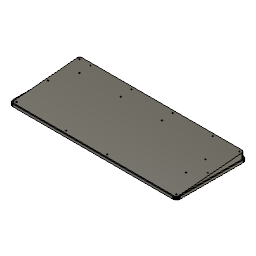
Base (Autodesk Fusion 360 design; units mm, degrees)
part number: 2026-06-20-14-02-00-105
Autodesk Fusion 360 part; units mm, degrees
note: some values were not read from the file. Chosen so that the rebuilt part matches the saved one: which pieces of a blend or face edit are solid.
(part 1 of 4)
imported_body "Derived Base Feature1" makes body 1
sketch "Sketch1" plane through (0, 0, 0) normal (0, 0, 1) x (1, 0, 0)
  line L0 (324.2389, -5.001) -> (324.612, -5.015)
  line L1 (324.612, -5.015) -> (324.9851, -5.059)
  line L2 (324.9851, -5.059) -> (325.3502, -5.132)
  line L3 (325.3502, -5.132) -> (325.71, -5.234)
  line L4 (325.71, -5.234) -> (326.0619, -5.363)
  line L5 (326.0619, -5.363) -> (326.4006, -5.52)
  line L6 (326.4006, -5.52) -> (326.726, -5.702)
  line L7 (326.726, -5.702) -> (327.0382, -5.91)
  line L8 (327.0382, -5.91) -> (327.3319, -6.142)
  line L9 (327.3319, -6.142) -> (327.6071, -6.395)
  line L10 (327.6071, -6.395) -> (327.8611, -6.67)
  line L11 (327.8611, -6.67) -> (328.0913, -6.964)
  line L12 (328.0913, -6.964) -> (328.3003, -7.275)
  line L13 (328.3003, -7.275) -> (328.4829, -7.601)
  line L14 (328.4829, -7.601) -> (328.639, -7.94)
  line L15 (328.639, -7.94) -> (328.7686, -8.291)
  line L16 (328.7686, -8.291) -> (328.8691, -8.651)
  line L17 (328.8691, -8.651) -> (328.9432, -9.018)
  line L18 (328.9432, -9.018) -> (328.9882, -9.389)
  line L19 (328.9882, -9.389) -> (329.0014, -9.763)
  line L20 (329.0014, -9.763) -> (329.0014, -133.7389)
  line L21 (329.0014, -133.7389) -> (328.9882, -134.1131)
  line L22 (328.9882, -134.1131) -> (328.9432, -134.484)
  line L23 (328.9432, -134.484) -> (328.8691, -134.851)
  line L24 (328.8691, -134.851) -> (328.7686, -135.2111)
  line L25 (328.7686, -135.2111) -> (328.639, -135.5619)
  line L26 (328.639, -135.5619) -> (328.4829, -135.9011)
  line L27 (328.4829, -135.9011) -> (328.3003, -136.2271)
  line L28 (328.3003, -136.2271) -> (328.0913, -136.538)
  line L29 (328.0913, -136.538) -> (327.8611, -136.8319)
  line L30 (327.8611, -136.8319) -> (327.6071, -137.1071)
  line L31 (327.6071, -137.1071) -> (327.3319, -137.36)
  line L32 (327.3319, -137.36) -> (327.0382, -137.5921)
  line L33 (327.0382, -137.5921) -> (326.726, -137.8)
  line L34 (326.726, -137.8) -> (326.4006, -137.9821)
  line L35 (326.4006, -137.9821) -> (326.0619, -138.139)
  line L36 (326.0619, -138.139) -> (325.71, -138.2681)
  line L37 (325.71, -138.2681) -> (325.3502, -138.3699)
  line L38 (325.3502, -138.3699) -> (324.9851, -138.443)
  line L39 (324.9851, -138.443) -> (324.612, -138.4869)
  line L40 (324.612, -138.4869) -> (324.2389, -138.502)
  line L41 (324.2389, -138.502) -> (9.763, -138.5009)
  line L42 (9.763, -138.5009) -> (9.389, -138.4869)
  line L43 (9.389, -138.4869) -> (9.018, -138.443)
  line L44 (9.018, -138.443) -> (8.651, -138.3699)
  line L45 (8.651, -138.3699) -> (8.291, -138.2681)
  line L46 (8.291, -138.2681) -> (7.94, -138.139)
  line L47 (7.94, -138.139) -> (7.601, -137.9821)
  line L48 (7.601, -137.9821) -> (7.275, -137.8)
  line L49 (7.275, -137.8) -> (6.964, -137.5921)
  line L50 (6.964, -137.5921) -> (6.67, -137.36)
  line L51 (6.67, -137.36) -> (6.395, -137.1071)
  line L52 (6.395, -137.1071) -> (6.142, -136.8319)
  line L53 (6.142, -136.8319) -> (5.91, -136.538)
  line L54 (5.91, -136.538) -> (5.702, -136.2271)
  line L55 (5.702, -136.2271) -> (5.52, -135.9011)
  line L56 (5.52, -135.9011) -> (5.363, -135.5619)
  line L57 (5.363, -135.5619) -> (5.234, -135.2111)
  line L58 (5.234, -135.2111) -> (5.132, -134.851)
  line L59 (5.132, -134.851) -> (5.059, -134.484)
  line L60 (5.059, -134.484) -> (5.015, -134.1131)
  line L61 (5.015, -134.1131) -> (5, -133.7389)
  line L62 (5, -133.7389) -> (5.001, -9.763)
  line L63 (5.001, -9.763) -> (5.015, -9.389)
  line L64 (5.015, -9.389) -> (5.059, -9.018)
  line L65 (5.059, -9.018) -> (5.132, -8.651)
  line L66 (5.132, -8.651) -> (5.234, -8.291)
  line L67 (5.234, -8.291) -> (5.363, -7.94)
  line L68 (5.363, -7.94) -> (5.52, -7.601)
  line L69 (5.52, -7.601) -> (5.702, -7.275)
  line L70 (5.702, -7.275) -> (5.91, -6.964)
  line L71 (5.91, -6.964) -> (6.142, -6.67)
  line L72 (6.142, -6.67) -> (6.395, -6.395)
  line L73 (6.395, -6.395) -> (6.67, -6.142)
  line L74 (6.67, -6.142) -> (6.964, -5.91)
  line L75 (6.964, -5.91) -> (7.275, -5.702)
  line L76 (7.275, -5.702) -> (7.601, -5.52)
  line L77 (7.601, -5.52) -> (7.94, -5.363)
  line L78 (7.94, -5.363) -> (8.291, -5.234)
  line L79 (8.291, -5.234) -> (8.651, -5.132)
  line L80 (8.651, -5.132) -> (9.018, -5.059)
  line L81 (9.018, -5.059) -> (9.389, -5.015)
  line L82 (9.389, -5.015) -> (9.763, -5)
  line L83 (9.763, -5) -> (324.2389, -5.001)
  line L84 (324.2654, -5.0281) -> (324.6411, -5.0421)
  line L85 (324.6411, -5.0421) -> (325.0115, -5.0861)
  line L86 (325.0115, -5.0861) -> (325.3793, -5.1591)
  line L87 (325.3793, -5.1591) -> (325.7391, -5.2611)
  line L88 (325.7391, -5.2611) -> (326.0884, -5.3901)
  line L89 (326.0884, -5.3901) -> (326.427, -5.5471)
  line L90 (326.427, -5.5471) -> (326.7551, -5.7291)
  line L91 (326.7551, -5.7291) -> (327.0647, -5.9371)
  line L92 (327.0647, -5.9371) -> (327.3584, -6.1691)
  line L93 (327.3584, -6.1691) -> (327.6336, -6.4221)
  line L94 (327.6336, -6.4221) -> (327.8875, -6.6971)
  line L95 (327.8875, -6.6971) -> (328.1204, -6.9911)
  line L96 (328.1204, -6.9911) -> (328.3268, -7.3021)
  line L97 (328.3268, -7.3021) -> (328.5093, -7.6281)
  line L98 (328.5093, -7.6281) -> (328.6654, -7.9671)
  line L99 (328.6654, -7.9671) -> (328.795, -8.3181)
  line L100 (328.795, -8.3181) -> (328.8982, -8.6781)
  line L101 (328.8982, -8.6781) -> (328.9697, -9.0451)
  line L102 (328.9697, -9.0451) -> (329.0147, -9.4161)
  line L103 (329.0147, -9.4161) -> (329.0279, -9.7901)
  line L104 (329.0279, -9.7901) -> (329.0279, -133.7662)
  line L105 (329.0279, -133.7662) -> (329.0147, -134.14)
  line L106 (329.0147, -134.14) -> (328.9697, -134.511)
  line L107 (328.9697, -134.511) -> (328.8982, -134.878)
  line L108 (328.8982, -134.878) -> (328.795, -135.2381)
  line L109 (328.795, -135.2381) -> (328.6654, -135.5892)
  line L110 (328.6654, -135.5892) -> (328.5093, -135.9281)
  line L111 (328.5093, -135.9281) -> (328.3268, -136.2541)
  line L112 (328.3268, -136.2541) -> (328.1204, -136.565)
  line L113 (328.1204, -136.565) -> (327.8875, -136.8592)
  line L114 (327.8875, -136.8592) -> (327.6336, -137.1341)
  line L115 (327.6336, -137.1341) -> (327.3584, -137.387)
  line L116 (327.3584, -137.387) -> (327.0647, -137.6191)
  line L117 (327.0647, -137.6191) -> (326.7551, -137.827)
  line L118 (326.7551, -137.827) -> (326.427, -138.0091)
  line L119 (326.427, -138.0091) -> (326.0884, -138.1662)
  line L120 (326.0884, -138.1662) -> (325.7391, -138.2951)
  line L121 (325.7391, -138.2951) -> (325.3793, -138.3972)
  line L122 (325.3793, -138.3972) -> (325.0115, -138.47)
  line L123 (325.0115, -138.47) -> (324.6411, -138.5141)
  line L124 (324.6411, -138.5141) -> (324.2654, -138.5289)
  line L125 (324.2654, -138.5289) -> (9.7901, -138.5282)
  line L126 (9.7901, -138.5282) -> (9.4161, -138.5141)
  line L127 (9.4161, -138.5141) -> (9.0451, -138.47)
  line L128 (9.0451, -138.47) -> (8.6781, -138.3972)
  line L129 (8.6781, -138.3972) -> (8.3181, -138.2951)
  line L130 (8.3181, -138.2951) -> (7.9671, -138.1662)
  line L131 (7.9671, -138.1662) -> (7.6281, -138.0091)
  line L132 (7.6281, -138.0091) -> (7.3021, -137.827)
  line L133 (7.3021, -137.827) -> (6.9911, -137.6191)
  line L134 (6.9911, -137.6191) -> (6.6971, -137.387)
  line L135 (6.6971, -137.387) -> (6.4221, -137.1341)
  line L136 (6.4221, -137.1341) -> (6.1691, -136.8592)
  line L137 (6.1691, -136.8592) -> (5.9371, -136.565)
  line L138 (5.9371, -136.565) -> (5.7291, -136.2541)
  line L139 (5.7291, -136.2541) -> (5.5471, -135.9281)
  line L140 (5.5471, -135.9281) -> (5.3901, -135.5892)
  line L141 (5.3901, -135.5892) -> (5.2611, -135.2381)
  line L142 (5.2611, -135.2381) -> (5.1591, -134.878)
  line L143 (5.1591, -134.878) -> (5.0861, -134.511)
  line L144 (5.0861, -134.511) -> (5.0421, -134.14)
  line L145 (5.0421, -134.14) -> (5.0271, -133.7662)
  line L146 (5.0271, -133.7662) -> (5.0281, -9.7901)
  line L147 (5.0281, -9.7901) -> (5.0421, -9.4161)
  line L148 (5.0421, -9.4161) -> (5.0861, -9.0451)
  line L149 (5.0861, -9.0451) -> (5.1591, -8.6781)
  line L150 (5.1591, -8.6781) -> (5.2611, -8.3181)
  line L151 (5.2611, -8.3181) -> (5.3901, -7.9671)
  line L152 (5.3901, -7.9671) -> (5.5471, -7.6281)
  line L153 (5.5471, -7.6281) -> (5.7291, -7.3021)
  line L154 (5.7291, -7.3021) -> (5.9371, -6.9911)
  line L155 (5.9371, -6.9911) -> (6.1691, -6.6971)
  line L156 (6.1691, -6.6971) -> (6.4221, -6.4221)
  line L157 (6.4221, -6.4221) -> (6.6971, -6.1691)
  line L158 (6.6971, -6.1691) -> (6.9911, -5.9371)
  line L159 (6.9911, -5.9371) -> (7.3021, -5.7291)
  line L160 (7.3021, -5.7291) -> (7.6281, -5.5471)
  line L161 (7.6281, -5.5471) -> (7.9671, -5.3901)
  line L162 (7.9671, -5.3901) -> (8.3181, -5.2611)
  line L163 (8.3181, -5.2611) -> (8.6781, -5.1591)
  line L164 (8.6781, -5.1591) -> (9.0451, -5.0861)
  line L165 (9.0451, -5.0861) -> (9.4161, -5.0421)
  line L166 (9.4161, -5.0421) -> (9.7901, -5.0271)
  line L167 (9.7901, -5.0271) -> (324.2654, -5.0281)
  line L168 (9.9401, -9.9401) -> (9.9401, -133.6162)
  line L169 (9.9401, -133.6162) -> (324.1172, -133.6162)
  line L170 (324.1172, -133.6162) -> (324.1172, -9.9401)
  line L171 (324.1172, -9.9401) -> (9.9401, -9.9401)
  line L172 (8.9397, -4.5648) -> (9.3495, -4.5162)
  line L173 (9.3495, -4.5162) -> (9.753, -4.5)
  line L174 (9.753, -4.5) -> (324.2483, -4.501)
  line L175 (324.2483, -4.501) -> (324.6507, -4.5161)
  line L176 (324.6507, -4.5161) -> (325.0635, -4.5648)
  line L177 (325.0635, -4.5648) -> (325.4676, -4.6456)
  line L178 (325.4676, -4.6456) -> (325.8645, -4.7581)
  line L179 (325.8645, -4.7581) -> (326.2534, -4.9007)
  line L180 (326.2534, -4.9007) -> (326.6281, -5.0744)
  line L181 (326.6281, -5.0744) -> (326.987, -5.2751)
  line L182 (326.987, -5.2751) -> (327.3323, -5.5051)
  line L183 (327.3323, -5.5051) -> (327.6566, -5.7613)
  line L184 (327.6566, -5.7613) -> (327.9605, -6.0408)
  line L185 (327.9605, -6.0408) -> (328.2422, -6.3457)
  line L186 (328.2422, -6.3457) -> (328.4962, -6.67)
  line L187 (328.4962, -6.67) -> (328.7266, -7.013)
  line L188 (328.7266, -7.013) -> (328.9288, -7.3739)
  line L189 (328.9288, -7.3739) -> (329.1012, -7.7485)
  line L190 (329.1012, -7.7485) -> (329.2447, -8.1369)
  line L191 (329.2447, -8.1369) -> (329.3556, -8.5341)
  line L192 (329.3556, -8.5341) -> (329.4372, -8.9383)
  line L193 (329.4372, -8.9383) -> (329.4872, -9.35)
  line L194 (329.4872, -9.35) -> (329.5014, -9.7542)
  line L195 (329.5014, -9.7542) -> (329.5014, -133.7478)
  line L196 (329.5014, -133.7478) -> (329.4872, -134.1521)
  line L197 (329.4872, -134.1521) -> (329.4372, -134.5637)
  line L198 (329.4372, -134.5637) -> (329.3556, -134.9678)
  line L199 (329.3556, -134.9678) -> (329.2447, -135.3652)
  line L200 (329.2447, -135.3652) -> (329.1013, -135.7534)
  line L201 (329.1013, -135.7534) -> (328.9288, -136.1282)
  line L202 (328.9288, -136.1282) -> (328.7266, -136.4892)
  line L203 (328.7266, -136.4892) -> (328.4961, -136.832)
  line L204 (328.4961, -136.832) -> (328.2422, -137.1562)
  line L205 (328.2422, -137.1562) -> (327.9606, -137.4613)
  line L206 (327.9606, -137.4613) -> (327.6566, -137.7408)
  line L207 (327.6566, -137.7408) -> (327.3323, -137.997)
  line L208 (327.3323, -137.997) -> (326.987, -138.2269)
  line L209 (326.987, -138.2269) -> (326.6281, -138.4277)
  line L210 (326.6281, -138.4277) -> (326.2534, -138.6013)
  line L211 (326.2534, -138.6013) -> (325.8645, -138.744)
  line L212 (325.8645, -138.744) -> (325.4675, -138.8564)
  line L213 (325.4675, -138.8564) -> (325.0635, -138.9372)
  line L214 (325.0635, -138.9372) -> (324.6514, -138.9857)
  line L215 (324.6514, -138.9857) -> (324.249, -139.002)
  line L216 (324.249, -139.002) -> (9.7536, -139.0009)
  line L217 (9.7536, -139.0009) -> (9.3502, -138.9858)
  line L218 (9.3502, -138.9858) -> (8.9397, -138.9372)
  line L219 (8.9397, -138.9372) -> (8.534, -138.8565)
  line L220 (8.534, -138.8565) -> (8.1364, -138.744)
  line L221 (8.1364, -138.744) -> (7.7484, -138.6012)
  line L222 (7.7484, -138.6012) -> (7.3738, -138.4279)
  line L223 (7.3738, -138.4279) -> (7.0137, -138.2268)
  line L224 (7.0137, -138.2268) -> (6.6697, -137.9968)
  line L225 (6.6697, -137.9968) -> (6.3454, -137.7408)
  line L226 (6.3454, -137.7408) -> (6.0411, -137.4609)
  line L227 (6.0411, -137.4609) -> (5.7612, -137.1565)
  line L228 (5.7612, -137.1565) -> (5.5054, -136.8323)
  line L229 (5.5054, -136.8323) -> (5.2752, -136.4884)
  line L230 (5.2752, -136.4884) -> (5.0742, -136.1283)
  line L231 (5.0742, -136.1283) -> (4.9007, -135.7535)
  line L232 (4.9007, -135.7535) -> (4.7581, -135.3657)
  line L233 (4.7581, -135.3657) -> (4.6455, -134.9681)
  line L234 (4.6455, -134.9681) -> (4.5648, -134.5623)
  line L235 (4.5648, -134.5623) -> (4.5162, -134.1526)
  line L236 (4.5162, -134.1526) -> (4.5, -133.749)
  line L237 (4.5, -133.749) -> (4.501, -9.7536)
  line L238 (4.501, -9.7536) -> (4.5161, -9.3501)
  line L239 (4.5161, -9.3501) -> (4.5648, -8.9397)
  line L240 (4.5648, -8.9397) -> (4.6455, -8.5339)
  line L241 (4.6455, -8.5339) -> (4.7581, -8.1364)
  line L242 (4.7581, -8.1364) -> (4.9007, -7.7484)
  line L243 (4.9007, -7.7484) -> (5.0742, -7.3738)
  line L244 (5.0742, -7.3738) -> (5.2752, -7.0137)
  line L245 (5.2752, -7.0137) -> (5.5053, -6.6697)
  line L246 (5.5053, -6.6697) -> (5.7612, -6.3454)
  line L247 (5.7612, -6.3454) -> (6.0411, -6.0411)
  line L248 (6.0411, -6.0411) -> (6.3454, -5.7612)
  line L249 (6.3454, -5.7612) -> (6.6697, -5.5053)
  line L250 (6.6697, -5.5053) -> (7.0137, -5.2752)
  line L251 (7.0137, -5.2752) -> (7.3737, -5.0742)
  line L252 (7.3737, -5.0742) -> (7.7484, -4.9007)
  line L253 (7.7484, -4.9007) -> (8.1364, -4.7581)
  line L254 (8.1364, -4.7581) -> (8.5339, -4.6455)
  line L255 (8.5339, -4.6455) -> (8.9397, -4.5648)
  line L256 (6.4647, -3.2911) -> (6.9819, -3.0516)
  line L257 (6.9819, -3.0516) -> (7.5179, -2.8546)
  line L258 (7.5179, -2.8546) -> (8.0654, -2.6995)
  line L259 (8.0654, -2.6995) -> (8.6263, -2.5879)
  line L260 (8.6263, -2.5879) -> (9.1914, -2.5209)
  line L261 (9.1914, -2.5209) -> (9.7129, -2.5)
  line L262 (9.7129, -2.5) -> (324.2858, -2.501)
  line L263 (324.2858, -2.501) -> (324.8056, -2.5205)
  line L264 (324.8056, -2.5205) -> (325.3772, -2.5879)
  line L265 (325.3772, -2.5879) -> (325.9371, -2.6999)
  line L266 (325.9371, -2.6999) -> (326.4823, -2.8544)
  line L267 (326.4823, -2.8544) -> (327.0195, -3.0513)
  line L268 (327.0195, -3.0513) -> (327.5381, -3.2918)
  line L269 (327.5381, -3.2918) -> (328.0311, -3.5675)
  line L270 (328.0311, -3.5675) -> (328.5085, -3.8855)
  line L271 (328.5085, -3.8855) -> (328.9551, -4.2384)
  line L272 (328.9551, -4.2384) -> (329.3743, -4.6238)
  line L273 (329.3743, -4.6238) -> (329.7667, -5.0485)
  line L274 (329.7667, -5.0485) -> (330.1156, -5.4942)
  line L275 (330.1156, -5.4942) -> (330.4319, -5.9649)
  line L276 (330.4319, -5.9649) -> (330.7124, -6.4656)
  line L277 (330.7124, -6.4656) -> (330.9504, -6.9827)
  line L278 (330.9504, -6.9827) -> (331.149, -7.5204)
  line L279 (331.149, -7.5204) -> (331.3016, -8.0666)
  line L280 (331.3016, -8.0666) -> (331.4132, -8.6195)
  line L281 (331.4132, -8.6195) -> (331.4829, -9.194)
  line L282 (331.4829, -9.194) -> (331.5014, -9.7189)
  line L283 (331.5014, -9.7189) -> (331.5014, -133.7831)
  line L284 (331.5014, -133.7831) -> (331.4829, -134.308)
  line L285 (331.4829, -134.308) -> (331.4132, -134.8825)
  line L286 (331.4132, -134.8825) -> (331.3016, -135.4353)
  line L287 (331.3016, -135.4353) -> (331.149, -135.9818)
  line L288 (331.149, -135.9818) -> (330.9504, -136.5192)
  line L289 (330.9504, -136.5192) -> (330.7125, -137.0363)
  line L290 (330.7125, -137.0363) -> (330.4317, -137.5375)
  line L291 (330.4317, -137.5375) -> (330.1155, -138.008)
  line L292 (330.1155, -138.008) -> (329.7669, -138.4531)
  line L293 (329.7669, -138.4531) -> (329.3745, -138.8782)
  line L294 (329.3745, -138.8782) -> (328.9551, -139.2637)
  line L295 (328.9551, -139.2637) -> (328.5085, -139.6166)
  line L296 (328.5085, -139.6166) -> (328.0312, -139.9345)
  line L297 (328.0312, -139.9345) -> (327.5379, -140.2104)
  line L298 (327.5379, -140.2104) -> (327.0196, -140.4505)
  line L299 (327.0196, -140.4505) -> (326.4822, -140.6477)
  line L300 (326.4822, -140.6477) -> (325.9367, -140.8021)
  line L301 (325.9367, -140.8021) -> (325.377, -140.9141)
  line L302 (325.377, -140.9141) -> (324.8089, -140.981)
  line L303 (324.8089, -140.981) -> (324.2894, -141.002)
  line L304 (324.2894, -141.002) -> (9.7161, -141.0009)
  line L305 (9.7161, -141.0009) -> (9.1949, -140.9814)
  line L306 (9.1949, -140.9814) -> (8.6265, -140.9141)
  line L307 (8.6265, -140.9141) -> (8.0658, -140.8025)
  line L308 (8.0658, -140.8025) -> (7.5179, -140.6475)
  line L309 (7.5179, -140.6475) -> (6.9818, -140.4503)
  line L310 (6.9818, -140.4503) -> (6.4649, -140.211)
  line L311 (6.4649, -140.211) -> (5.9687, -139.9339)
  line L312 (5.9687, -139.9339) -> (5.4925, -139.6155)
  line L313 (5.4925, -139.6155) -> (5.047, -139.2639)
  line L314 (5.047, -139.2639) -> (4.6255, -138.8762)
  line L315 (4.6255, -138.8762) -> (4.2379, -138.4547)
  line L316 (4.2379, -138.4547) -> (3.8868, -138.0098)
  line L317 (3.8868, -138.0098) -> (3.5682, -137.5337)
  line L318 (3.5682, -137.5337) -> (3.291, -137.0371)
  line L319 (3.291, -137.0371) -> (3.0516, -136.52)
  line L320 (3.0516, -136.52) -> (2.8546, -135.9843)
  line L321 (2.8546, -135.9843) -> (2.6995, -135.4364)
  line L322 (2.6995, -135.4364) -> (2.5879, -134.8757)
  line L323 (2.5879, -134.8757) -> (2.5209, -134.3107)
  line L324 (2.5209, -134.3107) -> (2.5, -133.789)
  line L325 (2.5, -133.789) -> (2.501, -9.7162)
  line L326 (2.501, -9.7162) -> (2.5205, -9.1947)
  line L327 (2.5205, -9.1947) -> (2.5879, -8.6263)
  line L328 (2.5879, -8.6263) -> (2.6995, -8.0655)
  line L329 (2.6995, -8.0655) -> (2.8546, -7.5179)
  line L330 (2.8546, -7.5179) -> (3.0516, -6.9819)
  line L331 (3.0516, -6.9819) -> (3.2911, -6.4648)
  line L332 (3.2911, -6.4648) -> (3.5681, -5.9687)
  line L333 (3.5681, -5.9687) -> (3.8866, -5.4925)
  line L334 (3.8866, -5.4925) -> (4.2381, -5.047)
  line L335 (4.2381, -5.047) -> (4.6257, -4.6257)
  line L336 (4.6257, -4.6257) -> (5.047, -4.2381)
  line L337 (5.047, -4.2381) -> (5.4925, -3.8866)
  line L338 (5.4925, -3.8866) -> (5.9687, -3.5681)
  line L339 (5.9687, -3.5681) -> (6.4647, -3.2911)
  dimension "d1" = -0.5
  dimension "d2" = -2
extrude "Extrude2" add sketch "Sketch1" along normal blind 1.5 separate body contours L172 L173 L174 L175 L176 L177 L178 L179 L180 L181 L182 L183 L184 L185 L186 L187 L188 L189 L190 L191 L192 L193 L194 L195 L196 L197 L198 L199 L200 L201 L202 L203 L204 L205 L206 L207 L208 L209 L210 L211 L212 L213 L214 L215 L216 L217 L218 L219 L220 L221 L222 L223 L224 L225 L226 L227 L228 L229 L230 L231 L232 L233 L234 L235 L236 L237 L238 L239 L240 L241 L242 L243 L244 L245 L246 L247 L248 L249 L250 L251 L252 L253 L254 L255 makes body 2
extrude "Extrude3" add sketch "Sketch1" along normal blind 1.5 separate body contours L10 L11 L12 L13 L14 L15 L16 L17 L18 L19 L20 L21 L22 L23 L24 L25 L26 L27 L28 L29 L30 L31 L32 L33 L34 L35 L36 L37 L38 L39 L40 L41 L42 L43 L44 L45 L46 L47 L48 L49 L50 L51 L52 L84 L85 L86 L87 L88 L89 L90 L91 L92 L93 L94 L135 L136 L137 L138 L139 L140 L141 L142 L143 L144 L145 L146 L147 L148 L149 L150 L151 L152 L153 L154 L155 L156 L157 L158 L159 L160 L161 L162 L163 L164 L165 L166 L167 | L168 L169 L170 L171 makes body 3
extrude "Extrude4" add sketch "Sketch1" along normal blind 1.5 contours L256 L257 L258 L259 L260 L261 L262 L263 L264 L265 L266 L267 L268 L269 L270 L271 L272 L273 L274 L275 L276 L277 L278 L279 L280 L281 L282 L283 L284 L285 L286 L287 L288 L289 L290 L291 L292 L293 L294 L295 L296 L297 L298 L299 L300 L301 L302 L303 L304 L305 L306 L307 L308 L309 L310 L311 L312 L313 L314 L315 L316 L317 L318 L319 L320 L321 L322 L323 L324 L325 L326 L327 L328 L329 L330 L331 L332 L333 L334 L335 L336 L337 L338 L339 bodies 2
sketch "Sketch2" plane through (-138.3507, 57.5384, 7.01) normal (0, 0, 1) x (-1, 0, 0)
  line L0 (-462.8147, 62.7033) -> (-462.439, 62.6893)
  line L1 (-462.439, 62.6893) -> (-148.1137, 62.6883)
  line L2 (-148.1137, 62.6883) -> (-147.7397, 62.7033)
  line L3 (-147.7397, 62.7033) -> (-147.3687, 62.7473)
  line L4 (-147.3687, 62.7473) -> (-147.0017, 62.8203)
  line L5 (-147.0017, 62.8203) -> (-146.6417, 62.9223)
  line L6 (-146.6417, 62.9223) -> (-146.2907, 63.0513)
  line L7 (-146.2907, 63.0513) -> (-145.9517, 63.2083)
  line L8 (-145.9517, 63.2083) -> (-145.6257, 63.3903)
  line L9 (-145.6257, 63.3903) -> (-145.3147, 63.5983)
  line L10 (-145.3147, 63.5983) -> (-145.0207, 63.8303)
  line L11 (-145.0207, 63.8303) -> (-144.7457, 64.0833)
  line L12 (-144.7457, 64.0833) -> (-144.4927, 64.3583)
  line L13 (-144.4927, 64.3583) -> (-144.2607, 64.6523)
  line L14 (-144.2607, 64.6523) -> (-144.0527, 64.9633)
  line L15 (-144.0527, 64.9633) -> (-143.8707, 65.2893)
  line L16 (-143.8707, 65.2893) -> (-143.7137, 65.6283)
  line L17 (-143.7137, 65.6283) -> (-143.5847, 65.9793)
  line L18 (-143.5847, 65.9793) -> (-143.4827, 66.3393)
  line L19 (-143.4827, 66.3393) -> (-143.4097, 66.7063)
  line L20 (-143.4097, 66.7063) -> (-143.3657, 67.0773)
  line L21 (-143.3657, 67.0773) -> (-143.3517, 67.4513)
  line L22 (-143.3517, 67.4513) -> (-143.3507, 191.2773)
  line L23 (-143.3507, 191.2773) -> (-143.3657, 191.6512)
  line L24 (-143.3657, 191.6512) -> (-143.4097, 192.0224)
  line L25 (-143.4097, 192.0224) -> (-143.4827, 192.3894)
  line L26 (-143.4827, 192.3894) -> (-143.5847, 192.7492)
  line L27 (-143.5847, 192.7492) -> (-143.7137, 193.1003)
  line L28 (-143.7137, 193.1003) -> (-143.8707, 193.4392)
  line L29 (-143.8707, 193.4392) -> (-144.0527, 193.7652)
  line L30 (-144.0527, 193.7652) -> (-144.2607, 194.0764)
  line L31 (-144.2607, 194.0764) -> (-144.4927, 194.3703)
  line L32 (-144.4927, 194.3703) -> (-144.7457, 194.6452)
  line L33 (-144.7457, 194.6452) -> (-145.0207, 194.8984)
  line L34 (-145.0207, 194.8984) -> (-145.3147, 195.1302)
  line L35 (-145.3147, 195.1302) -> (-145.6257, 195.3382)
  line L36 (-145.6257, 195.3382) -> (-145.9517, 195.5202)
  line L37 (-145.9517, 195.5202) -> (-146.2907, 195.6774)
  line L38 (-146.2907, 195.6774) -> (-146.6417, 195.8062)
  line L39 (-146.6417, 195.8062) -> (-147.0017, 195.9083)
  line L40 (-147.0017, 195.9083) -> (-147.3687, 195.9814)
  line L41 (-147.3687, 195.9814) -> (-147.7397, 196.0253)
  line L42 (-147.7397, 196.0253) -> (-148.1137, 196.0404)
  line L43 (-148.1137, 196.0404) -> (-462.439, 196.0404)
  line L44 (-462.439, 196.0404) -> (-462.8147, 196.0253)
  line L45 (-462.8147, 196.0253) -> (-463.1851, 195.9814)
  line L46 (-463.1851, 195.9814) -> (-463.5528, 195.9083)
  line L47 (-463.5528, 195.9083) -> (-463.9127, 195.8062)
  line L48 (-463.9127, 195.8062) -> (-464.2619, 195.6774)
  line L49 (-464.2619, 195.6774) -> (-464.6006, 195.5202)
  line L50 (-464.6006, 195.5202) -> (-464.9287, 195.3382)
  line L51 (-464.9287, 195.3382) -> (-465.2382, 195.1302)
  line L52 (-465.2382, 195.1302) -> (-465.532, 194.8984)
  line L53 (-465.532, 194.8984) -> (-465.8071, 194.6452)
  line L54 (-465.8071, 194.6452) -> (-466.0611, 194.3703)
  line L55 (-466.0611, 194.3703) -> (-466.2939, 194.0764)
  line L56 (-466.2939, 194.0764) -> (-466.5003, 193.7652)
  line L57 (-466.5003, 193.7652) -> (-466.6829, 193.4392)
  line L58 (-466.6829, 193.4392) -> (-466.839, 193.1003)
  line L59 (-466.839, 193.1003) -> (-466.9686, 192.7492)
  line L60 (-466.9686, 192.7492) -> (-467.0718, 192.3894)
  line L61 (-467.0718, 192.3894) -> (-467.1433, 192.0224)
  line L62 (-467.1433, 192.0224) -> (-467.1882, 191.6512)
  line L63 (-467.1882, 191.6512) -> (-467.2014, 191.2773)
  line L64 (-467.2014, 191.2773) -> (-467.2014, 67.4513)
  line L65 (-467.2014, 67.4513) -> (-467.1882, 67.0773)
  line L66 (-467.1882, 67.0773) -> (-467.1433, 66.7063)
  line L67 (-467.1433, 66.7063) -> (-467.0718, 66.3393)
  line L68 (-467.0718, 66.3393) -> (-466.9686, 65.9793)
  line L69 (-466.9686, 65.9793) -> (-466.839, 65.6283)
  line L70 (-466.839, 65.6283) -> (-466.6829, 65.2893)
  line L71 (-466.6829, 65.2893) -> (-466.5003, 64.9633)
  line L72 (-466.5003, 64.9633) -> (-466.2939, 64.6523)
  line L73 (-466.2939, 64.6523) -> (-466.0611, 64.3583)
  line L74 (-466.0611, 64.3583) -> (-465.8071, 64.0833)
  line L75 (-465.8071, 64.0833) -> (-465.532, 63.8303)
  line L76 (-465.532, 63.8303) -> (-465.2382, 63.5983)
  line L77 (-465.2382, 63.5983) -> (-464.9287, 63.3903)
  line L78 (-464.9287, 63.3903) -> (-464.6006, 63.2083)
  line L79 (-464.6006, 63.2083) -> (-464.2619, 63.0513)
  line L80 (-464.2619, 63.0513) -> (-463.9127, 62.9223)
  line L81 (-463.9127, 62.9223) -> (-463.5528, 62.8203)
  line L82 (-463.5528, 62.8203) -> (-463.1851, 62.7473)
  line L83 (-463.1851, 62.7473) -> (-462.8147, 62.7033)
  circle A0 centre (-148.1139, 191.2768) radius 1.1
  arc A1 (-158.9635, 180.5254) -> (-158.2763, 181.2126) centre (-158.703, 180.9521) ccw
  arc A2 (-158.9635, 180.5254) -> (-159.1198, 180.5693) centre (-159.1198, 180.2696) ccw
  line L84 (-159.1198, 180.5693) -> (-160.0202, 180.5693)
  line L85 (-160.0202, 180.5693) -> (-160.9206, 180.5693)
  arc A3 (-160.9206, 180.5693) -> (-161.0769, 180.5254) centre (-160.9206, 180.2693) ccw
  arc A4 (-161.7641, 181.2126) -> (-161.0769, 180.5254) centre (-161.3374, 180.9521) ccw
  arc A5 (-161.7641, 181.2126) -> (-161.7202, 181.3689) centre (-162.0202, 181.3689) ccw
  line L86 (-161.7202, 181.3689) -> (-161.7202, 182.0693)
  line L87 (-161.7202, 182.0693) -> (-161.7202, 182.7696)
  arc A6 (-161.7202, 182.7696) -> (-161.7641, 182.9259) centre (-162.0202, 182.7696) ccw
  arc A7 (-161.0769, 183.6132) -> (-161.7641, 182.9259) centre (-161.3374, 183.1864) ccw
  arc A8 (-161.0769, 183.6132) -> (-160.9206, 183.5693) centre (-160.9206, 183.8693) ccw
  line L88 (-160.9206, 183.5693) -> (-160.0202, 183.5693)
  line L89 (-160.0202, 183.5693) -> (-159.1198, 183.5693)
  arc A9 (-159.1198, 183.5693) -> (-158.9635, 183.6132) centre (-159.1199, 183.8693) ccw
  arc A10 (-158.2763, 182.9259) -> (-158.9635, 183.6132) centre (-158.703, 183.1864) ccw
  arc A11 (-158.2763, 182.9259) -> (-158.3202, 182.7696) centre (-158.0201, 182.7696) ccw
  line L90 (-158.3202, 182.7696) -> (-158.3202, 182.0693)
  line L91 (-158.3202, 182.0693) -> (-158.3202, 181.3689)
  arc A12 (-158.3202, 181.3689) -> (-158.2763, 181.2126) centre (-158.0201, 181.3689) ccw
  circle A13 centre (-154.9402, 176.9893) radius 0.875
  circle A14 centre (-160.0202, 176.9893) radius 1.9939
  circle A15 centre (-165.1002, 176.9893) radius 0.875
  arc A16 (-182.776, 180.5254) -> (-182.0888, 181.2126) centre (-182.5155, 180.9521) ccw
  arc A17 (-182.776, 180.5254) -> (-182.9323, 180.5693) centre (-182.9323, 180.2696) ccw
  line L92 (-182.9323, 180.5693) -> (-183.8327, 180.5693)
  line L93 (-183.8327, 180.5693) -> (-184.7331, 180.5693)
  arc A18 (-184.7331, 180.5693) -> (-184.8894, 180.5254) centre (-184.7331, 180.2693) ccw
  arc A19 (-185.5766, 181.2126) -> (-184.8894, 180.5254) centre (-185.1499, 180.9521) ccw
  arc A20 (-185.5766, 181.2126) -> (-185.5327, 181.3689) centre (-185.8327, 181.3689) ccw
  line L94 (-185.5327, 181.3689) -> (-185.5327, 182.0693)
  line L95 (-185.5327, 182.0693) -> (-185.5327, 182.7696)
  arc A21 (-185.5327, 182.7696) -> (-185.5766, 182.9259) centre (-185.8327, 182.7696) ccw
  arc A22 (-184.8894, 183.6132) -> (-185.5766, 182.9259) centre (-185.1499, 183.1864) ccw
  arc A23 (-184.8894, 183.6132) -> (-184.7331, 183.5693) centre (-184.7331, 183.8693) ccw
  line L96 (-184.7331, 183.5693) -> (-183.8327, 183.5693)
  line L97 (-183.8327, 183.5693) -> (-182.9323, 183.5693)
  arc A24 (-182.9323, 183.5693) -> (-182.776, 183.6132) centre (-182.9324, 183.8693) ccw
  arc A25 (-182.0888, 182.9259) -> (-182.776, 183.6132) centre (-182.5155, 183.1864) ccw
  arc A26 (-182.0888, 182.9259) -> (-182.1327, 182.7696) centre (-181.8326, 182.7696) ccw
  line L98 (-182.1327, 182.7696) -> (-182.1327, 182.0693)
  line L99 (-182.1327, 182.0693) -> (-182.1327, 181.3689)
  arc A27 (-182.1327, 181.3689) -> (-182.0888, 181.2126) centre (-181.8326, 181.3689) ccw
  circle A28 centre (-178.7527, 176.9893) radius 0.875
  circle A29 centre (-183.8327, 176.9893) radius 1.9939
  circle A30 centre (-188.9127, 176.9893) radius 0.875
  circle A31 centre (-202.5652, 176.9893) radius 0.875
  arc A32 (-206.5885, 180.5254) -> (-205.9013, 181.2126) centre (-206.328, 180.9521) ccw
  arc A33 (-206.5885, 180.5254) -> (-206.7448, 180.5693) centre (-206.7448, 180.2696) ccw
  line L100 (-206.7448, 180.5693) -> (-207.6452, 180.5693)
  line L101 (-207.6452, 180.5693) -> (-208.5456, 180.5693)
  arc A34 (-208.5456, 180.5693) -> (-208.7019, 180.5254) centre (-208.5456, 180.2693) ccw
  arc A35 (-209.3891, 181.2126) -> (-208.7019, 180.5254) centre (-208.9624, 180.9521) ccw
  arc A36 (-209.3891, 181.2126) -> (-209.3452, 181.3689) centre (-209.6452, 181.3689) ccw
  line L102 (-209.3452, 181.3689) -> (-209.3452, 182.0693)
  line L103 (-209.3452, 182.0693) -> (-209.3452, 182.7696)
  arc A37 (-209.3452, 182.7696) -> (-209.3891, 182.9259) centre (-209.6452, 182.7696) ccw
  arc A38 (-208.7019, 183.6132) -> (-209.3891, 182.9259) centre (-208.9624, 183.1864) ccw
  arc A39 (-208.7019, 183.6132) -> (-208.5456, 183.5693) centre (-208.5456, 183.8693) ccw
  line L104 (-208.5456, 183.5693) -> (-207.6452, 183.5693)
  line L105 (-207.6452, 183.5693) -> (-206.7448, 183.5693)
  arc A40 (-206.7448, 183.5693) -> (-206.5885, 183.6132) centre (-206.7449, 183.8693) ccw
  arc A41 (-205.9013, 182.9259) -> (-206.5885, 183.6132) centre (-206.328, 183.1864) ccw
  arc A42 (-205.9013, 182.9259) -> (-205.9452, 182.7696) centre (-205.6451, 182.7696) ccw
  line L106 (-205.9452, 182.7696) -> (-205.9452, 182.0693)
  line L107 (-205.9452, 182.0693) -> (-205.9452, 181.3689)
  arc A43 (-205.9452, 181.3689) -> (-205.9013, 181.2126) centre (-205.6451, 181.3689) ccw
  circle A44 centre (-207.6452, 176.9893) radius 1.9939
  circle A45 centre (-212.7252, 176.9893) radius 0.875
  circle A46 centre (-156.2102, 174.4493) radius 1.5
  circle A47 centre (-162.5602, 171.9093) radius 1.5
  circle A48 centre (-180.0227, 174.4493) radius 1.5
  circle A49 centre (-186.3727, 171.9093) radius 1.5
  arc A50 (-168.4885, 161.4754) -> (-167.8013, 162.1626) centre (-168.228, 161.9021) ccw
  arc A51 (-168.4885, 161.4754) -> (-168.6448, 161.5193) centre (-168.6448, 161.2196) ccw
  line L108 (-168.6448, 161.5193) -> (-169.5452, 161.5193)
  line L109 (-169.5452, 161.5193) -> (-170.4456, 161.5193)
  arc A52 (-170.4456, 161.5193) -> (-170.6019, 161.4754) centre (-170.4456, 161.2193) ccw
  arc A53 (-171.2891, 162.1626) -> (-170.6019, 161.4754) centre (-170.8624, 161.9021) ccw
  arc A54 (-171.2891, 162.1626) -> (-171.2452, 162.3189) centre (-171.5452, 162.3189) ccw
  line L110 (-171.2452, 162.3189) -> (-171.2452, 163.0193)
  line L111 (-171.2452, 163.0193) -> (-171.2452, 163.7196)
  arc A55 (-171.2452, 163.7196) -> (-171.2891, 163.8759) centre (-171.5452, 163.7196) ccw
  arc A56 (-170.6019, 164.5632) -> (-171.2891, 163.8759) centre (-170.8624, 164.1364) ccw
  arc A57 (-170.6019, 164.5632) -> (-170.4456, 164.5193) centre (-170.4456, 164.8193) ccw
  line L112 (-170.4456, 164.5193) -> (-169.5452, 164.5193)
  line L113 (-169.5452, 164.5193) -> (-168.6448, 164.5193)
  arc A58 (-168.6448, 164.5193) -> (-168.4885, 164.5632) centre (-168.6449, 164.8193) ccw
  arc A59 (-167.8013, 163.8759) -> (-168.4885, 164.5632) centre (-168.228, 164.1364) ccw
  arc A60 (-167.8013, 163.8759) -> (-167.8452, 163.7196) centre (-167.5451, 163.7196) ccw
  line L114 (-167.8452, 163.7196) -> (-167.8452, 163.0193)
  line L115 (-167.8452, 163.0193) -> (-167.8452, 162.3189)
  arc A61 (-167.8452, 162.3189) -> (-167.8013, 162.1626) centre (-167.5451, 162.3189) ccw
  circle A62 centre (-203.8352, 174.4493) radius 1.5
  circle A63 centre (-210.1852, 171.9093) radius 1.5
  arc A64 (-199.4448, 161.4754) -> (-198.7575, 162.1626) centre (-199.1843, 161.9021) ccw
  arc A65 (-199.4448, 161.4754) -> (-199.6011, 161.5193) centre (-199.601, 161.2196) ccw
  line L116 (-199.6011, 161.5193) -> (-200.5014, 161.5193)
  line L117 (-200.5014, 161.5193) -> (-201.4018, 161.5193)
  arc A66 (-201.4018, 161.5193) -> (-201.5581, 161.4754) centre (-201.4018, 161.2193) ccw
  arc A67 (-202.2454, 162.1626) -> (-201.5581, 161.4754) centre (-201.8186, 161.9021) ccw
  arc A68 (-202.2454, 162.1626) -> (-202.2014, 162.3189) centre (-202.5014, 162.3189) ccw
  line L118 (-202.2014, 162.3189) -> (-202.2014, 163.0193)
  line L119 (-202.2014, 163.0193) -> (-202.2014, 163.7196)
  arc A69 (-202.2014, 163.7196) -> (-202.2454, 163.8759) centre (-202.5014, 163.7196) ccw
  arc A70 (-201.5581, 164.5632) -> (-202.2454, 163.8759) centre (-201.8186, 164.1364) ccw
  arc A71 (-201.5581, 164.5632) -> (-201.4018, 164.5193) centre (-201.4018, 164.8193) ccw
  line L120 (-201.4018, 164.5193) -> (-200.5014, 164.5193)
  line L121 (-200.5014, 164.5193) -> (-199.6011, 164.5193)
  arc A72 (-199.6011, 164.5193) -> (-199.4448, 164.5632) centre (-199.6011, 164.8193) ccw
  arc A73 (-198.7575, 163.8759) -> (-199.4448, 164.5632) centre (-199.1843, 164.1364) ccw
  arc A74 (-198.7575, 163.8759) -> (-198.8014, 163.7196) centre (-198.5014, 163.7196) ccw
  line L122 (-198.8014, 163.7196) -> (-198.8014, 163.0193)
  line L123 (-198.8014, 163.0193) -> (-198.8014, 162.3189)
  arc A75 (-198.8014, 162.3189) -> (-198.7575, 162.1626) centre (-198.5014, 162.3189) ccw
  arc A76 (-218.4948, 161.4754) -> (-217.8075, 162.1626) centre (-218.2343, 161.9021) ccw
  arc A77 (-218.4948, 161.4754) -> (-218.6511, 161.5193) centre (-218.651, 161.2196) ccw
  line L124 (-218.6511, 161.5193) -> (-219.5514, 161.5193)
  line L125 (-219.5514, 161.5193) -> (-220.4518, 161.5193)
  arc A78 (-220.4518, 161.5193) -> (-220.6081, 161.4754) centre (-220.4518, 161.2193) ccw
  arc A79 (-221.2954, 162.1626) -> (-220.6081, 161.4754) centre (-220.8686, 161.9021) ccw
  arc A80 (-221.2954, 162.1626) -> (-221.2514, 162.3189) centre (-221.5514, 162.3189) ccw
  line L126 (-221.2514, 162.3189) -> (-221.2514, 163.0193)
  line L127 (-221.2514, 163.0193) -> (-221.2514, 163.7196)
  arc A81 (-221.2514, 163.7196) -> (-221.2954, 163.8759) centre (-221.5514, 163.7196) ccw
  arc A82 (-220.6081, 164.5632) -> (-221.2954, 163.8759) centre (-220.8686, 164.1364) ccw
  arc A83 (-220.6081, 164.5632) -> (-220.4518, 164.5193) centre (-220.4518, 164.8193) ccw
  line L128 (-220.4518, 164.5193) -> (-219.5514, 164.5193)
  line L129 (-219.5514, 164.5193) -> (-218.6511, 164.5193)
  arc A84 (-218.6511, 164.5193) -> (-218.4948, 164.5632) centre (-218.6511, 164.8193) ccw
  arc A85 (-217.8075, 163.8759) -> (-218.4948, 164.5632) centre (-218.2343, 164.1364) ccw
  arc A86 (-217.8075, 163.8759) -> (-217.8514, 163.7196) centre (-217.5514, 163.7196) ccw
  line L130 (-217.8514, 163.7196) -> (-217.8514, 163.0193)
  line L131 (-217.8514, 163.0193) -> (-217.8514, 162.3189)
  arc A87 (-217.8514, 162.3189) -> (-217.8075, 162.1626) centre (-217.5514, 162.3189) ccw
  circle A88 centre (-245.7452, 191.2768) radius 1.1
  arc A89 (-280.8266, 181.2126) -> (-280.1394, 180.5254) centre (-280.3999, 180.9521) ccw
  arc A90 (-280.8266, 181.2126) -> (-280.7827, 181.3689) centre (-281.0827, 181.3689) ccw
  line L132 (-280.7827, 181.3689) -> (-280.7827, 182.0693)
  line L133 (-280.7827, 182.0693) -> (-280.7827, 182.7696)
  arc A91 (-280.7827, 182.7696) -> (-280.8266, 182.9259) centre (-281.0827, 182.7696) ccw
  arc A92 (-280.1394, 183.6132) -> (-280.8266, 182.9259) centre (-280.3999, 183.1864) ccw
  arc A93 (-280.1394, 183.6132) -> (-279.9831, 183.5693) centre (-279.9831, 183.8693) ccw
  line L134 (-279.9831, 183.5693) -> (-279.0827, 183.5693)
  line L135 (-279.0827, 183.5693) -> (-278.1823, 183.5693)
  arc A94 (-278.1823, 183.5693) -> (-278.026, 183.6132) centre (-278.1824, 183.8693) ccw
  arc A95 (-277.3388, 182.9259) -> (-278.026, 183.6132) centre (-277.7655, 183.1864) ccw
  arc A96 (-277.3388, 182.9259) -> (-277.3827, 182.7696) centre (-277.0826, 182.7696) ccw
  line L136 (-277.3827, 182.7696) -> (-277.3827, 182.0693)
  line L137 (-277.3827, 182.0693) -> (-277.3827, 181.3689)
  arc A97 (-277.3827, 181.3689) -> (-277.3388, 181.2126) centre (-277.0826, 181.3689) ccw
  arc A98 (-278.026, 180.5254) -> (-277.3388, 181.2126) centre (-277.7655, 180.9521) ccw
  arc A99 (-278.026, 180.5254) -> (-278.1823, 180.5693) centre (-278.1823, 180.2696) ccw
  line L138 (-278.1823, 180.5693) -> (-279.0827, 180.5693)
  line L139 (-279.0827, 180.5693) -> (-279.9831, 180.5693)
  arc A100 (-279.9831, 180.5693) -> (-280.1394, 180.5254) centre (-279.9831, 180.2693) ccw
  circle A101 centre (-274.0027, 176.9893) radius 0.875
  circle A102 centre (-279.0827, 176.9893) radius 1.9939
  circle A103 centre (-284.1627, 176.9893) radius 0.875
  arc A104 (-237.5448, 161.4754) -> (-236.8575, 162.1626) centre (-237.2843, 161.9021) ccw
  arc A105 (-237.5448, 161.4754) -> (-237.7011, 161.5193) centre (-237.701, 161.2196) ccw
  line L140 (-237.7011, 161.5193) -> (-238.6014, 161.5193)
  line L141 (-238.6014, 161.5193) -> (-239.5018, 161.5193)
  arc A106 (-239.5018, 161.5193) -> (-239.6581, 161.4754) centre (-239.5018, 161.2193) ccw
  arc A107 (-240.3454, 162.1626) -> (-239.6581, 161.4754) centre (-239.9186, 161.9021) ccw
  arc A108 (-240.3454, 162.1626) -> (-240.3014, 162.3189) centre (-240.6014, 162.3189) ccw
  line L142 (-240.3014, 162.3189) -> (-240.3014, 163.0193)
  line L143 (-240.3014, 163.0193) -> (-240.3014, 163.7196)
  arc A109 (-240.3014, 163.7196) -> (-240.3454, 163.8759) centre (-240.6014, 163.7196) ccw
  arc A110 (-239.6581, 164.5632) -> (-240.3454, 163.8759) centre (-239.9186, 164.1364) ccw
  arc A111 (-239.6581, 164.5632) -> (-239.5018, 164.5193) centre (-239.5018, 164.8193) ccw
  line L144 (-239.5018, 164.5193) -> (-238.6014, 164.5193)
  line L145 (-238.6014, 164.5193) -> (-237.7011, 164.5193)
  arc A112 (-237.7011, 164.5193) -> (-237.5448, 164.5632) centre (-237.7011, 164.8193) ccw
  arc A113 (-236.8575, 163.8759) -> (-237.5448, 164.5632) centre (-237.2843, 164.1364) ccw
  arc A114 (-236.8575, 163.8759) -> (-236.9014, 163.7196) centre (-236.6014, 163.7196) ccw
  line L146 (-236.9014, 163.7196) -> (-236.9014, 163.0193)
  line L147 (-236.9014, 163.0193) -> (-236.9014, 162.3189)
  arc A115 (-236.9014, 162.3189) -> (-236.8575, 162.1626) centre (-236.6014, 162.3189) ccw
  arc A116 (-256.5948, 161.4754) -> (-255.9075, 162.1626) centre (-256.3343, 161.9021) ccw
  arc A117 (-256.5948, 161.4754) -> (-256.7511, 161.5193) centre (-256.751, 161.2196) ccw
  line L148 (-256.7511, 161.5193) -> (-257.6514, 161.5193)
  line L149 (-257.6514, 161.5193) -> (-258.5518, 161.5193)
  arc A118 (-258.5518, 161.5193) -> (-258.7081, 161.4754) centre (-258.5518, 161.2193) ccw
  arc A119 (-259.3954, 162.1626) -> (-258.7081, 161.4754) centre (-258.9686, 161.9021) ccw
  arc A120 (-259.3954, 162.1626) -> (-259.3514, 162.3189) centre (-259.6514, 162.3189) ccw
  line L150 (-259.3514, 162.3189) -> (-259.3514, 163.0193)
  line L151 (-259.3514, 163.0193) -> (-259.3514, 163.7196)
  arc A121 (-259.3514, 163.7196) -> (-259.3954, 163.8759) centre (-259.6514, 163.7196) ccw
  arc A122 (-258.7081, 164.5632) -> (-259.3954, 163.8759) centre (-258.9686, 164.1364) ccw
  arc A123 (-258.7081, 164.5632) -> (-258.5518, 164.5193) centre (-258.5518, 164.8193) ccw
  line L152 (-258.5518, 164.5193) -> (-257.6514, 164.5193)
  line L153 (-257.6514, 164.5193) -> (-256.7511, 164.5193)
  arc A124 (-256.7511, 164.5193) -> (-256.5948, 164.5632) centre (-256.7511, 164.8193) ccw
  arc A125 (-255.9075, 163.8759) -> (-256.5948, 164.5632) centre (-256.3343, 164.1364) ccw
  arc A126 (-255.9075, 163.8759) -> (-255.9514, 163.7196) centre (-255.6514, 163.7196) ccw
  line L154 (-255.9514, 163.7196) -> (-255.9514, 163.0193)
  line L155 (-255.9514, 163.0193) -> (-255.9514, 162.3189)
  arc A127 (-255.9514, 162.3189) -> (-255.9075, 162.1626) centre (-255.6514, 162.3189) ccw
  circle A128 centre (-275.2727, 174.4493) radius 1.5
  circle A129 centre (-281.6227, 171.9093) radius 1.5
  arc A130 (-275.6448, 161.4754) -> (-274.9575, 162.1626) centre (-275.3843, 161.9021) ccw
  arc A131 (-275.6448, 161.4754) -> (-275.8011, 161.5193) centre (-275.801, 161.2196) ccw
  line L156 (-275.8011, 161.5193) -> (-276.7014, 161.5193)
  line L157 (-276.7014, 161.5193) -> (-277.6018, 161.5193)
  arc A132 (-277.6018, 161.5193) -> (-277.7581, 161.4754) centre (-277.6018, 161.2193) ccw
  arc A133 (-278.4454, 162.1626) -> (-277.7581, 161.4754) centre (-278.0186, 161.9021) ccw
  arc A134 (-278.4454, 162.1626) -> (-278.4014, 162.3189) centre (-278.7014, 162.3189) ccw
  line L158 (-278.4014, 162.3189) -> (-278.4014, 163.0193)
  line L159 (-278.4014, 163.0193) -> (-278.4014, 163.7196)
  arc A135 (-278.4014, 163.7196) -> (-278.4454, 163.8759) centre (-278.7014, 163.7196) ccw
  arc A136 (-277.7581, 164.5632) -> (-278.4454, 163.8759) centre (-278.0186, 164.1364) ccw
  arc A137 (-277.7581, 164.5632) -> (-277.6018, 164.5193) centre (-277.6018, 164.8193) ccw
  line L160 (-277.6018, 164.5193) -> (-276.7014, 164.5193)
  line L161 (-276.7014, 164.5193) -> (-275.8011, 164.5193)
  arc A138 (-275.8011, 164.5193) -> (-275.6448, 164.5632) centre (-275.8011, 164.8193) ccw
  arc A139 (-274.9575, 163.8759) -> (-275.6448, 164.5632) centre (-275.3843, 164.1364) ccw
  arc A140 (-274.9575, 163.8759) -> (-275.0014, 163.7196) centre (-274.7014, 163.7196) ccw
  line L162 (-275.0014, 163.7196) -> (-275.0014, 163.0193)
  line L163 (-275.0014, 163.0193) -> (-275.0014, 162.3189)
  arc A141 (-275.0014, 162.3189) -> (-274.9575, 162.1626) centre (-274.7014, 162.3189) ccw
  arc A142 (-297.4954, 162.1626) -> (-296.8081, 161.4754) centre (-297.0686, 161.9021) ccw
  arc A143 (-297.4954, 162.1626) -> (-297.4514, 162.3189) centre (-297.7514, 162.3189) ccw
  line L164 (-297.4514, 162.3189) -> (-297.4514, 163.0193)
  line L165 (-297.4514, 163.0193) -> (-297.4514, 163.7196)
  arc A144 (-297.4514, 163.7196) -> (-297.4954, 163.8759) centre (-297.7514, 163.7196) ccw
  arc A145 (-296.8081, 164.5632) -> (-297.4954, 163.8759) centre (-297.0686, 164.1364) ccw
  arc A146 (-296.8081, 164.5632) -> (-296.6518, 164.5193) centre (-296.6518, 164.8193) ccw
  line L166 (-296.6518, 164.5193) -> (-295.7514, 164.5193)
  line L167 (-295.7514, 164.5193) -> (-294.8511, 164.5193)
  arc A147 (-294.8511, 164.5193) -> (-294.6948, 164.5632) centre (-294.8511, 164.8193) ccw
  arc A148 (-294.0075, 163.8759) -> (-294.6948, 164.5632) centre (-294.4343, 164.1364) ccw
  arc A149 (-294.0075, 163.8759) -> (-294.0514, 163.7196) centre (-293.7514, 163.7196) ccw
  line L168 (-294.0514, 163.7196) -> (-294.0514, 163.0193)
  line L169 (-294.0514, 163.0193) -> (-294.0514, 162.3189)
  arc A150 (-294.0514, 162.3189) -> (-294.0075, 162.1626) centre (-293.7514, 162.3189) ccw
  arc A151 (-294.6948, 161.4754) -> (-294.0075, 162.1626) centre (-294.4343, 161.9021) ccw
  arc A152 (-294.6948, 161.4754) -> (-294.8511, 161.5193) centre (-294.851, 161.2196) ccw
  line L170 (-294.8511, 161.5193) -> (-295.7514, 161.5193)
  line L171 (-295.7514, 161.5193) -> (-296.6518, 161.5193)
  arc A153 (-296.6518, 161.5193) -> (-296.8081, 161.4754) centre (-296.6518, 161.2193) ccw
  circle A154 centre (-164.4652, 157.9393) radius 0.875
  circle A155 centre (-165.7352, 155.3993) radius 1.5
  circle A156 centre (-169.5452, 157.9393) radius 1.9939
  circle A157 centre (-174.6252, 157.9393) radius 0.875
  circle A158 centre (-172.0852, 152.8593) radius 1.5
  circle A159 centre (-195.4214, 157.9393) radius 0.875
  circle A160 centre (-200.5014, 157.9393) radius 1.9939
  circle A161 centre (-205.5814, 157.9393) radius 0.875
  circle A162 centre (-196.6914, 155.3993) radius 1.5
  circle A163 centre (-203.0414, 152.8593) radius 1.5
  circle A164 centre (-214.4714, 157.9393) radius 0.875
  circle A165 centre (-219.5514, 157.9393) radius 1.9939
  circle A166 centre (-224.6314, 157.9393) radius 0.875
  circle A167 centre (-215.7414, 155.3993) radius 1.5
  circle A168 centre (-222.0914, 152.8593) radius 1.5
  arc A169 (-163.726, 142.4254) -> (-163.0388, 143.1126) centre (-163.4655, 142.8521) ccw
  arc A170 (-163.726, 142.4254) -> (-163.8823, 142.4693) centre (-163.8823, 142.1696) ccw
  line L172 (-163.8823, 142.4693) -> (-164.7827, 142.4693)
  line L173 (-164.7827, 142.4693) -> (-165.6831, 142.4693)
  arc A171 (-165.6831, 142.4693) -> (-165.8394, 142.4254) centre (-165.6831, 142.1693) ccw
  arc A172 (-166.5266, 143.1126) -> (-165.8394, 142.4254) centre (-166.0999, 142.8521) ccw
  arc A173 (-166.5266, 143.1126) -> (-166.4827, 143.2689) centre (-166.7827, 143.2689) ccw
  line L174 (-166.4827, 143.2689) -> (-166.4827, 143.9693)
  line L175 (-166.4827, 143.9693) -> (-166.4827, 144.6696)
  arc A174 (-166.4827, 144.6696) -> (-166.5266, 144.8259) centre (-166.7827, 144.6696) ccw
  arc A175 (-165.8394, 145.5132) -> (-166.5266, 144.8259) centre (-166.0999, 145.0864) ccw
  arc A176 (-165.8394, 145.5132) -> (-165.6831, 145.4693) centre (-165.6831, 145.7693) ccw
  line L176 (-165.6831, 145.4693) -> (-164.7827, 145.4693)
  line L177 (-164.7827, 145.4693) -> (-163.8823, 145.4693)
  arc A177 (-163.8823, 145.4693) -> (-163.726, 145.5132) centre (-163.8824, 145.7693) ccw
  arc A178 (-163.0388, 144.8259) -> (-163.726, 145.5132) centre (-163.4655, 145.0864) ccw
  arc A179 (-163.0388, 144.8259) -> (-163.0827, 144.6696) centre (-162.7826, 144.6696) ccw
  line L178 (-163.0827, 144.6696) -> (-163.0827, 143.9693)
  line L179 (-163.0827, 143.9693) -> (-163.0827, 143.2689)
  arc A180 (-163.0827, 143.2689) -> (-163.0388, 143.1126) centre (-162.7826, 143.2689) ccw
  circle A181 centre (-159.7027, 138.8893) radius 0.875
  circle A182 centre (-164.7827, 138.8893) radius 1.9939
  circle A183 centre (-169.8627, 138.8893) radius 0.875
  circle A184 centre (-185.8964, 138.8893) radius 0.875
  circle A185 centre (-160.9727, 136.3493) radius 1.5
  circle A186 centre (-148.1139, 129.3643) radius 1.1
  circle A187 centre (-167.3227, 133.8093) radius 1.5
  arc A188 (-189.9198, 142.4254) -> (-189.2325, 143.1126) centre (-189.6593, 142.8521) ccw
  arc A189 (-189.9198, 142.4254) -> (-190.0761, 142.4693) centre (-190.076, 142.1696) ccw
  line L180 (-190.0761, 142.4693) -> (-190.9764, 142.4693)
  line L181 (-190.9764, 142.4693) -> (-191.8768, 142.4693)
  arc A190 (-191.8768, 142.4693) -> (-192.0331, 142.4254) centre (-191.8768, 142.1693) ccw
  arc A191 (-192.7204, 143.1126) -> (-192.0331, 142.4254) centre (-192.2936, 142.8521) ccw
  arc A192 (-192.7204, 143.1126) -> (-192.6764, 143.2689) centre (-192.9764, 143.2689) ccw
  line L182 (-192.6764, 143.2689) -> (-192.6764, 143.9693)
  line L183 (-192.6764, 143.9693) -> (-192.6764, 144.6696)
  arc A193 (-192.6764, 144.6696) -> (-192.7204, 144.8259) centre (-192.9764, 144.6696) ccw
  arc A194 (-192.0331, 145.5132) -> (-192.7204, 144.8259) centre (-192.2936, 145.0864) ccw
  arc A195 (-192.0331, 145.5132) -> (-191.8768, 145.4693) centre (-191.8768, 145.7693) ccw
  line L184 (-191.8768, 145.4693) -> (-190.9764, 145.4693)
  line L185 (-190.9764, 145.4693) -> (-190.0761, 145.4693)
  arc A196 (-190.0761, 145.4693) -> (-189.9198, 145.5132) centre (-190.0761, 145.7693) ccw
  arc A197 (-189.2325, 144.8259) -> (-189.9198, 145.5132) centre (-189.6593, 145.0864) ccw
  arc A198 (-189.2325, 144.8259) -> (-189.2764, 144.6696) centre (-188.9764, 144.6696) ccw
  line L186 (-189.2764, 144.6696) -> (-189.2764, 143.9693)
  line L187 (-189.2764, 143.9693) -> (-189.2764, 143.2689)
  arc A199 (-189.2764, 143.2689) -> (-189.2325, 143.1126) centre (-188.9764, 143.2689) ccw
  circle A200 centre (-190.9764, 138.8893) radius 1.9939
  circle A201 centre (-196.0564, 138.8893) radius 0.875
  circle A202 centre (-204.9464, 138.8893) radius 0.875
  arc A203 (-208.9698, 142.4254) -> (-208.2825, 143.1126) centre (-208.7093, 142.8521) ccw
  arc A204 (-208.9698, 142.4254) -> (-209.1261, 142.4693) centre (-209.126, 142.1696) ccw
  line L188 (-209.1261, 142.4693) -> (-210.0264, 142.4693)
  line L189 (-210.0264, 142.4693) -> (-210.9268, 142.4693)
  arc A205 (-210.9268, 142.4693) -> (-211.0831, 142.4254) centre (-210.9268, 142.1693) ccw
  arc A206 (-211.7704, 143.1126) -> (-211.0831, 142.4254) centre (-211.3436, 142.8521) ccw
  arc A207 (-211.7704, 143.1126) -> (-211.7264, 143.2689) centre (-212.0264, 143.2689) ccw
  line L190 (-211.7264, 143.2689) -> (-211.7264, 143.9693)
  line L191 (-211.7264, 143.9693) -> (-211.7264, 144.6696)
  arc A208 (-211.7264, 144.6696) -> (-211.7704, 144.8259) centre (-212.0264, 144.6696) ccw
  arc A209 (-211.0831, 145.5132) -> (-211.7704, 144.8259) centre (-211.3436, 145.0864) ccw
  arc A210 (-211.0831, 145.5132) -> (-210.9268, 145.4693) centre (-210.9268, 145.7693) ccw
  line L192 (-210.9268, 145.4693) -> (-210.0264, 145.4693)
  line L193 (-210.0264, 145.4693) -> (-209.1261, 145.4693)
  arc A211 (-209.1261, 145.4693) -> (-208.9698, 145.5132) centre (-209.1261, 145.7693) ccw
  arc A212 (-208.2825, 144.8259) -> (-208.9698, 145.5132) centre (-208.7093, 145.0864) ccw
  arc A213 (-208.2825, 144.8259) -> (-208.3264, 144.6696) centre (-208.0264, 144.6696) ccw
  line L194 (-208.3264, 144.6696) -> (-208.3264, 143.9693)
  line L195 (-208.3264, 143.9693) -> (-208.3264, 143.2689)
  arc A214 (-208.3264, 143.2689) -> (-208.2825, 143.1126) centre (-208.0264, 143.2689) ccw
  circle A215 centre (-210.0264, 138.8893) radius 1.9939
  circle A216 centre (-215.1064, 138.8893) radius 0.875
  circle A217 centre (-223.9964, 138.8893) radius 0.875
  circle A218 centre (-187.1664, 136.3493) radius 1.5
  circle A219 centre (-193.5164, 133.8093) radius 1.5
  circle A220 centre (-206.2164, 136.3493) radius 1.5
  circle A221 centre (-212.5664, 133.8093) radius 1.5